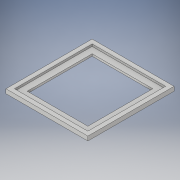
# Autodesk Inventor part: Scannframebottom
Saved by Autodesk Inventor 2019 (Build 230136000, 136)
## iProperties
Created: 2018-10-07
Part Number: Scannframebottom
Material: Generic
Document SubType Name: Modeling
Designer: paperspace
Density: 1 g/cm^3
Appearance: Default
Author: paperspace
Autodesk Inventor part; units mm, degrees
ref_plane "YZ Plane" through (0, 0, 0) normal (1, 0, 0) x (0, 1, 0)
ref_plane "XZ Plane" through (0, 0, 0) normal (0, 1, 0) x (-1, 0, 0)
ref_plane "XY Plane" through (0, 0, 0) normal (0, 0, 1) x (1, 0, 0)
sketch "Sketch1" plane through (0, 0, 0) normal (0, 1, 0) x (-1, 0, 0)
  point P0 (0, 0)
sketch "Sketch2" plane through (0, 0, 0) normal (0, 1, 0) x (-1, 0, 0)
  line L0 (0, 0) -> (57, 0)
  line L1 (57, 0) -> (57, -61)
  line L2 (57, -61) -> (0, -61)
  line L3 (0, -61) -> (0, 0)
  line L4 (67, -71) -> (67, 10)
  line L5 (67, 10) -> (-10, 10)
  line L6 (-10, 10) -> (-10, -71)
  line L7 (-10, -71) -> (67, -71)
  dimension "d0" = 57
  dimension "d1" = 61
  dimension "d2" = 10
  constraints: 16 end point, 4 parallel, 2 perpendicular, 1 horizontal, 3 other
  measures "d0" distance of L1.end L2.end
  measures "d1" distance of L0.end L1.end
  measures "d2" distance between parallel lines of L1 L4
extrude "Extrusion1" add sketch "Sketch2" along normal blind 2
sketch "Sketch3" plane through (0, 2, 0) normal (0, 1, 0) x (1, 0, 0)
  line L0 (10, -10) -> (10, 71) projected
  line L1 (-67, 71) -> (-67, -10) projected
  line L2 (10, -10) -> (-67, -10)
  line L3 (-67, -10) -> (-67, 71)
  line L4 (-67, 71) -> (10, 71)
  line L5 (10, 71) -> (10, -10)
  line L6 (6, 67) -> (-63, 67)
  line L7 (-63, 67) -> (-63, -6)
  line L8 (-63, -6) -> (6, -6)
  line L9 (6, -6) -> (6, 67)
  point P0 (0, 0)
  dimension "d5" = 4
  constraints: 16 end point, 4 parallel, 2 perpendicular, 1 horizontal, 3 other
  measures "d5" distance between parallel lines of L4 L6
extrude "Extrusion2" add sketch "Sketch3" along normal blind 2
body "Solid1"
